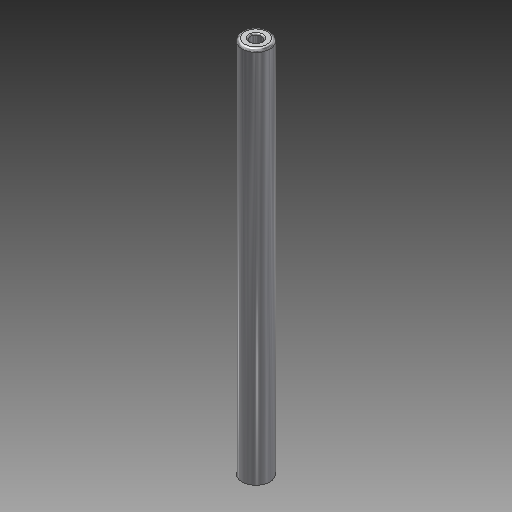
# Autodesk Inventor part: Nema 17 Shaft
Saved by Autodesk Inventor 2017 (Build 210142000, 142)
## iProperties
Created: 2015-09-21
Part Number: Nema 17 Shaft
Material: Stainless Steel
Document SubType Name: Modeling
Designer: Dr Kreigar
Density: 8 g/cm^3
Appearance: Semi-Polished
Mass: 10.4229 g
Surface Area: 11.6611 cm^2
Volume: 1.30287 cm^3
Author: Dr Kreigar
Autodesk Inventor part; units mm, degrees
ref_plane "YZ Plane" through (0, 0, 0) normal (1, 0, 0) x (0, 1, 0)
ref_plane "XZ Plane" through (0, 0, 0) normal (0, 1, 0) x (-1, 0, 0)
ref_plane "XY Plane" through (0, 0, 0) normal (0, 0, 1) x (1, 0, 0)
sketch "Sketch1" plane through (0, 0, 0) normal (0, 1, 0) x (-1, 0, 0)
  circle A0 centre (0, 0) radius 2.5
  dimension "d0" = 5
  constraints: 1 centre point, 1 coincident
  measures "d0" diameter of A0
extrude "Extrusion1" add sketch "Sketch1" along normal blind 68
fillet "Fillet1" radius 0.5 1 edges at (2.5, 68, 0)
hole "Hole1" at (0, 68, 0) direction (0, -1, 0) diameter 2 depth 10
fillet "Fillet2" radius 0.25 1 edges at (0, 68, -1)
body "Solid1"
